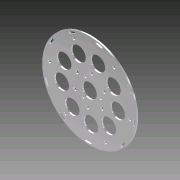
# Autodesk Inventor part: Traction Wheel Side Plate 1764
Saved by Autodesk Inventor 2011 (Build 150239000, 239)
## iProperties
Created: 2009-01-19
Part Number: Traction Wheel Side Plate 1764
Document SubType Name: Modeling
Designer: pmulligan
Density: 1 g/cm^3
Mass: 26.3519 g
Surface Area: 272.292 cm^2
Volume: 26.3519 cm^3
Author: pmulligan
Autodesk Inventor part; units mm, degrees
ref_plane "YZ Plane" through (0, 0, 0) normal (1, 0, 0) x (0, 1, 0)
ref_plane "XZ Plane" through (0, 0, 0) normal (0, 1, 0) x (-1, 0, 0)
ref_plane "XY Plane" through (0, 0, 0) normal (0, 0, 1) x (1, 0, 0)
sketch "Sketch1" plane through (0, 0, 0) normal (0, 0, 1) x (1, 0, 0)
  circle A0 centre (-11.7643, 11.3599) radius 71.8439
  circle A1 centre (-11.7643, 11.3599) radius 11.1125
  circle A2 centre (-18.3109, 26.8617) radius 2.032
  circle A3 centre (-21.916, -2.0606) radius 2.032
  circle A4 centre (4.9339, 9.2784) radius 2.032
  circle A5 centre (-33.7703, 2.1297) radius 2.4384
  circle A6 centre (-11.7643, 11.3599) radius 11.1125
  circle A7 centre (-14.7737, -12.3129) radius 2.4384
  circle A8 centre (-11.7643, 11.3599) radius 11.1125
  circle A9 centre (7.2322, -3.0827) radius 2.4384
  circle A10 centre (-11.7643, 11.3599) radius 11.1125
  circle A11 centre (10.2416, 20.5901) radius 2.4384
  circle A12 centre (-11.7643, 11.3599) radius 11.1125
  circle A13 centre (-8.755, 35.0327) radius 2.4384
  circle A14 centre (-11.7643, 11.3599) radius 11.1125
  circle A15 centre (-30.7609, 25.8024) radius 2.4384
  circle A16 centre (-28.6125, 51.2552) radius 11.1125
  circle A17 centre (-50.315, 31.0916) radius 11.1125
  circle A18 centre (-53.9792, 1.6954) radius 11.1125
  circle A19 centre (-37.8906, -23.1787) radius 11.1125
  circle A20 centre (-9.5772, -31.8919) radius 11.1125
  circle A21 centre (17.7128, -20.367) radius 11.1125
  circle A22 centre (31.2101, 6.0032) radius 11.1125
  circle A23 centre (24.5992, 34.8798) radius 11.1125
  circle A24 centre (0.9734, 52.7512) radius 11.1125
  circle A25 centre (-35.6556, 67.9328) radius 2.1654
  circle A26 centre (-72.7036, 18.9559) radius 2.1654
  circle A27 centre (-48.8123, -37.6171) radius 2.1654
  circle A28 centre (12.127, -45.2131) radius 2.1654
  circle A29 centre (49.1749, 3.7639) radius 2.1654
  circle A30 centre (25.2836, 60.3368) radius 2.1654
  line L0 (-11.7643, 11.3599) -> (-28.6125, 51.2552)
  line L1 (-28.6125, 51.2552) -> (-35.6556, 67.9328)
  line L2 (-35.6556, 67.9328) -> (-36.4981, 69.9276)
  line L3 (-36.4981, 69.9276) -> (-39.7145, 77.544)
  line L4 (-42.5987, 73.9272) -> (-35.111, 77.0893)
  line L5 (-34.0932, 74.6792) -> (-41.5809, 71.5171)
  arc A31 (-42.5987, 73.9272) -> (-41.5809, 71.5171) centre (-42.0898, 72.7221) ccw
  arc A32 (-34.0932, 74.6792) -> (-35.111, 77.0893) centre (-34.6021, 75.8843) ccw
  arc A33 (-1.1352, 80.2978) -> (-1.6838, 77.7398) centre (-1.4095, 79.0188) ccw
  line L6 (6.2634, 76.0353) -> (-1.6838, 77.7398)
  line L7 (-1.1352, 80.2978) -> (6.8121, 78.5933)
  arc A34 (6.2634, 76.0353) -> (6.8121, 78.5933) centre (6.5377, 77.3143) ccw
  arc A35 (-66.3735, 50.4207) -> (-68.5896, 51.8112) centre (-67.4816, 51.116) ccw
  line L8 (-66.3735, 50.4207) -> (-70.6934, 43.5357)
  arc A36 (-72.9095, 44.9262) -> (-70.6934, 43.5357) centre (-71.8014, 44.2309) ccw
  line L9 (-72.9095, 44.9262) -> (-68.5896, 51.8112)
  line L10 (-76.781, -13.904) -> (-79.2785, -6.1692)
  line L11 (-76.7888, -5.3654) -> (-74.2913, -13.1001)
  arc A37 (-76.7888, -5.3654) -> (-79.2785, -6.1692) centre (-78.0336, -5.7673) ccw
  arc A38 (-76.781, -13.904) -> (-74.2913, -13.1001) centre (-75.5361, -13.5021) ccw
  line L12 (-55.4361, -39.6371) -> (-48.9538, -44.5406)
  arc A39 (-50.5321, -46.6271) -> (-48.9538, -44.5406) centre (-49.7429, -45.5838) ccw
  line L13 (-50.5321, -46.6271) -> (-57.0144, -41.7236)
  arc A40 (-55.4361, -39.6371) -> (-57.0144, -41.7236) centre (-56.2252, -40.6804) ccw
  line L14 (-18.2875, -55.4635) -> (-10.1649, -55.7621)
  arc A41 (-10.2611, -58.3765) -> (-10.1649, -55.7621) centre (-10.213, -57.0693) ccw
  line L15 (-10.2611, -58.3765) -> (-18.3836, -58.0779)
  arc A42 (-18.2875, -55.4635) -> (-18.3836, -58.0779) centre (-18.3355, -56.7707) ccw
  line L16 (42.6231, -32.3142) -> (37.1734, -38.3445)
  line L17 (35.2324, -36.5904) -> (40.6821, -30.5601)
  arc A43 (42.6231, -32.3142) -> (40.6821, -30.5601) centre (41.6526, -31.4372) ccw
  arc A44 (35.2324, -36.5904) -> (37.1734, -38.3445) centre (36.2029, -37.4674) ccw
  arc A45 (54.2362, -0.9625) -> (56.8323, -1.2861) centre (55.5343, -1.1243) ccw
  line L18 (54.2362, -0.9625) -> (55.2416, 7.1031)
  line L19 (57.8377, 6.7795) -> (56.8323, -1.2861)
  arc A46 (57.8377, 6.7795) -> (55.2416, 7.1031) centre (56.5396, 6.9413) ccw
  arc A47 (49.368, 39.1224) -> (51.6802, 40.3464) centre (50.5241, 39.7344) ccw
  line L20 (49.368, 39.1224) -> (45.5653, 46.306)
  line L21 (47.8775, 47.53) -> (51.6802, 40.3464)
  arc A48 (47.8775, 47.53) -> (45.5653, 46.306) centre (46.7214, 46.918) ccw
  point P0 (-37.837, 73.0981)
  point P1 (2.2898, 76.8876)
  point P2 (-68.5334, 46.9782)
  point P3 (-75.5401, -9.2327)
  point P4 (-52.1949, -42.0889)
  point P5 (-14.2262, -55.6128)
  point P6 (37.9572, -33.5752)
  point P7 (54.7389, 3.0703)
  point P8 (47.4666, 42.7142)
  dimension "d20" = 143.6878
  dimension "d32" = 4.3307
  dimension "d21" = 22.225
  dimension "d22" = 4.064
  dimension "d23" = 3.683
  dimension "d24" = 360
  dimension "d25" = 4.8768
  dimension "d26" = 8.1026
  dimension "d27" = 10.3124
  dimension "d28" = 360
  dimension "d29" = 22.225
  dimension "d30" = 13.335
  dimension "d31" = 360
  dimension "d33" = 4.826
  dimension "d34" = 360
  dimension "d35" = 2.6162
  dimension "d36" = 4.826
  dimension "d37" = 35
  dimension "d38" = 35
  dimension "d39" = 50
  dimension "d40" = 70
  dimension "d41" = 50
  dimension "d42" = 70
  constraints: 47 centre point, 44 end point, 36 point on circle, 3 collinear, 1 coincident, 1 midpoint, 1 parallel, 1 perpendicular, 1 point on line, 164 other
  measures "d21" diameter of A1
  measures "d22" diameter of A2
  measures "d25" diameter of A5
  measures "d29" diameter of A16
  measures "d35" distance between parallel lines of L4 L5
  measures "d36" distance from line of L3.end L5
extrude "Extrusion1" add sketch "Sketch1" along normal blind 2.2225
body "Solid1"
